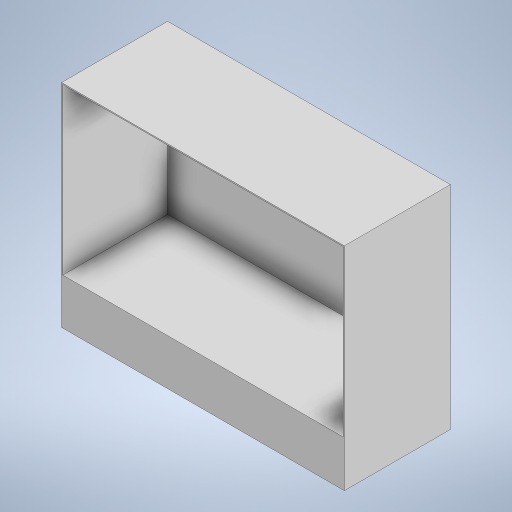
# Autodesk Inventor part: Top Bin
Saved by Autodesk Inventor 2024 (Build 280153000, 153)
## iProperties
Created: 2024-09-16
Part Number: Top Bin
Material: Generic
Document SubType Name: Modeling
Designer: srira
Density: 1 g/cm^3
Appearance: Default
Author: srira
Autodesk Inventor part; units mm, degrees
ref_plane "YZ Plane" through (0, 0, 0) normal (1, 0, 0) x (0, 1, 0)
ref_plane "XZ Plane" through (0, 0, 0) normal (0, 1, 0) x (-1, 0, 0)
ref_plane "XY Plane" through (0, 0, 0) normal (0, 0, 1) x (1, 0, 0)
sketch "Sketch1" plane through (0, 0, 0) normal (0, 0, 1) x (1, 0, 0)
  line L0 (-600, -450) -> (600, -450)
  line L1 (600, -450) -> (600, 450)
  line L2 (600, 450) -> (-600, 450)
  line L3 (-600, 450) -> (-600, -450)
  line L4 (-600, -450) -> (600, 450) construction
  line L5 (600, -450) -> (-600, 450) construction
  line L6 (-595, 445) -> (595, 445)
  line L7 (595, 445) -> (595, -255)
  line L8 (595, -255) -> (-595, -255)
  line L9 (-595, -255) -> (-595, 445)
  point P0 (0, 0)
  dimension "d0" = 1200
  dimension "d1" = 900
  dimension "d2" = 1190
  dimension "d3" = 700
  dimension "d4" = 5
  dimension "d5" = 5
  constraints: 20 end point, 4 parallel, 2 horizontal, 2 midpoint, 2 perpendicular
  measures "d0" distance of L2.end L1.end
  measures "d1" distance of L1.end L0.end
  measures "d2" distance of L7.end L8.end
  measures "d3" distance of L8.end L6.start
  measures "d4" distance between parallel lines of L3 L9
  measures "d5" distance between parallel lines of L2 L6
extrude "Extrusion1" add sketch "Sketch1" along normal blind 450
sketch "Sketch2" plane through (0, 0, 0) normal (0, 0, -1) x (-1, 0, 0)
  line L0 (-595, 445) -> (-595, -255) projected
  line L1 (595, -255) -> (595, 445) projected
  line L2 (-595, 445) -> (595, 445)
  line L3 (595, 445) -> (595, -255)
  line L4 (595, -255) -> (-595, -255)
  line L5 (-595, -255) -> (-595, 445)
  point P0 (0, 0)
  constraints: 8 end point, 2 parallel, 1 horizontal, 1 perpendicular
extrude "Extrusion2" add sketch "Sketch2" against normal blind 5
body "Solid1"
